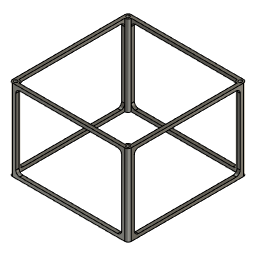
22.05.2024-Estructura electromagnet deslizante v1 (Autodesk Fusion 360 design; units mm, degrees)
Autodesk Fusion 360 part; units mm, degrees
note: some values were not read from the file. Set by a fixed rule: which sketch regions a step uses.
sketch "Sketch1" plane through (0, 0, 0) normal (0, 0, 1) x (1, 0, 0)
  line L0 (70, 70) -> (-70, 70)
  line L1 (-70, 70) -> (-70, -70)
  line L2 (-70, -70) -> (70, -70)
  line L3 (70, -70) -> (70, 70)
  line L4 (70, 70) -> (-70, -70) construction
  line L5 (-70, 70) -> (70, -70) construction
  line L6 (-74, 74) -> (-74, -74)
  line L7 (-74, -74) -> (74, -74)
  line L8 (74, -74) -> (74, 74)
  line L9 (74, 74) -> (-74, 74)
  circle A0 centre (70, 70) radius 4
  circle A1 centre (-70, 70) radius 4
  circle A2 centre (70, -70) radius 4
  circle A3 centre (-70, -70) radius 4
  dimension "d1" = 140
  dimension "d2" = 140
  dimension "d3" = 4
  dimension "d4" = 8
  dimension "d5" = 8
  dimension "d6" = 8
  constraint horizontal L0
  constraint perpendicular L0 L1
  constraint parallel L0 L2
  constraint parallel L1 L3
  constraint coincident L4 origin
  constraint coincident L5 origin
  constraint coincident L0.start L3.end
  constraint tangent L8 A0
  constraint coincident L0.end L1.start
  constraint coincident L2.end L3.start
  constraint coincident L1.end L2.start
  measures "d1" distance of L1.end L2.end
  measures "d2" distance of L0.end L1.end
  measures "d4" diameter of A1
  measures "d5" diameter of A2
  measures "d6" diameter of A3
extrude "Extrude1" add sketch "Sketch1" along normal blind 101 contours L0 L1 A1 | L0 L9 A0 A1 | L0 L1 A1 | L0 L3 A0 | L0 L3 A0 | L1 L6 A1 A3 | L3 L8 A0 A2 | L1 L2 A3 | L1 L2 A3 | L2 L3 A2 | L2 L3 A2 | L2 L7 A2 A3
sketch "Sketch2" plane through (0, -74, 0) normal (0, -1, 0) x (1, 0, 0)
  line L0 (-70, 0) -> (70, 0)
  line L1 (70, 0) -> (70, 101)
  line L2 (70, 101) -> (-70, 101)
  line L3 (-70, 101) -> (-70, 0)
  line L4 (-66, 101) -> (66, 101)
  line L5 (66, 101) -> (66, 0)
  line L6 (66, 0) -> (-66, 0)
  line L7 (-66, 0) -> (-66, 101)
  line L8 (62, 97) -> (62, 4)
  line L9 (62, 4) -> (-62, 4)
  line L10 (-62, 4) -> (-62, 97)
  line L11 (-62, 97) -> (62, 97)
  line L12 (66, 97) -> (-66, 97)
  line L13 (-66, 97) -> (-66, 4)
  line L14 (-66, 4) -> (66, 4)
  line L15 (66, 4) -> (66, 97)
  dimension "d9" = 4
  constraint horizontal L4
  constraint vertical L5
  constraint horizontal L6
  constraint vertical L7
  constraint coincident L0 L5.end
  constraint coincident L2 L4.start
  constraint horizontal L12
  constraint vertical L13
  constraint horizontal L14
  constraint vertical L15
  constraint coincident L7 L13.end
  constraint coincident L5 L12.start
extrude "Extrude2" cut sketch "Sketch2" against normal blind 4 contours L7 L10 L12 L13 L14 | L5 L8 L12 L14 L15 | L8 L9 L10 L11 L12 L14
sketch "Sketch3" plane through (-74, 0, 0) normal (-1, 0, 0) x (0, -1, 0)
  line L0 (-70, 0) -> (70, 0)
  line L1 (70, 0) -> (70, 101)
  line L2 (70, 101) -> (-70, 101)
  line L3 (-70, 101) -> (-70, 0)
  line L4 (66, 97) -> (-66, 97)
  line L5 (-66, 97) -> (-66, 4)
  line L6 (-66, 4) -> (66, 4)
  line L7 (66, 4) -> (66, 97)
  constraint horizontal L4
  constraint vertical L5
  constraint horizontal L6
  constraint vertical L7
extrude "Extrude3" cut sketch "Sketch3" against normal blind 4 contours L4 L5 L6 L7
sketch "Sketch4" plane through (0, 74, 0) normal (0, 1, 0) x (-1, 0, 0)
  line L0 (-70, 0) -> (70, 0)
  line L1 (70, 0) -> (70, 101)
  line L2 (70, 101) -> (-70, 101)
  line L3 (-70, 101) -> (-70, 0)
  line L4 (-66, 97) -> (66, 97)
  line L5 (66, 97) -> (66, 4)
  line L6 (66, 4) -> (-66, 4)
  line L7 (-66, 4) -> (-66, 97)
  constraint horizontal L4
  constraint vertical L5
  constraint horizontal L6
  constraint vertical L7
extrude "Extrude4" cut sketch "Sketch4" against normal blind 4 contours L4 L5 L6 L7
sketch "Sketch5" plane through (74, 0, 0) normal (1, 0, 0) x (0, 1, 0)
  line L0 (-70, 0) -> (70, 0)
  line L1 (70, 0) -> (70, 101)
  line L2 (70, 101) -> (-70, 101)
  line L3 (-70, 101) -> (-70, 0)
  line L4 (-66, 97) -> (66, 97)
  line L5 (66, 97) -> (66, 4)
  line L6 (66, 4) -> (-66, 4)
  line L7 (-66, 4) -> (-66, 97)
  constraint horizontal L4
  constraint vertical L5
  constraint horizontal L6
  constraint vertical L7
extrude "Extrude5" cut sketch "Sketch5" against normal blind 4 contours L4 L5 L6 L7
fillet "Fillet1" radius 5 4 edges at (66, -72, 97) (-66, -72, 97) (-66, -72, 4) (66, -72, 4)
fillet "Fillet2" radius 5 4 edges at (72, -66, 97) (72, 66, 97) (72, -66, 4) (72, 66, 4)
fillet "Fillet3" radius 5 4 edges at (66, 72, 97) (-66, 72, 97) (66, 72, 4) (-66, 72, 4)
fillet "Fillet4" radius 5 4 edges at (-72, 66, 97) (-72, -66, 97) (-72, 66, 4) (-72, -66, 4)
hole "Hole1" at (70, 70, 101) direction (0, 0, -1) diameter 4.25 depth 40 tip angle 118
hole "Hole2" at (70, -70, 101) direction (0, 0, -1) diameter 4.25 depth 40 tip angle 118
hole "Hole3" at (-70, -70, 101) direction (0, 0, -1) diameter 4.25 depth 40 tip angle 118
hole "Hole4" at (-70, 70, 101) direction (0, 0, -1) diameter 4.25 depth 40 tip angle 118
